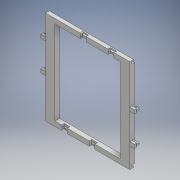
# Autodesk Inventor part: Male_Final
Saved by Autodesk Inventor 2017 (Build 210142000, 142)
## iProperties
Created: 2018-11-19
Part Number: Male_Final
Material: Generic
Document SubType Name: Modeling
Designer: Ralph
Density: 1 g/cm^3
Appearance: Default
Author: Ralph
Autodesk Inventor part; units mm, degrees
ref_plane "YZ Plane" through (0, 0, 0) normal (1, 0, 0) x (0, 1, 0)
ref_plane "XZ Plane" through (0, 0, 0) normal (0, 1, 0) x (-1, 0, 0)
ref_plane "XY Plane" through (0, 0, 0) normal (0, 0, 1) x (1, 0, 0)
sketch "Sketch1" plane through (0, 0, 0) normal (0, 1, 0) x (-1, 0, 0)
  line L0 (0, 0) -> (90, 0)
  line L1 (90, 0) -> (90, -100)
  line L2 (90, -100) -> (0, -100)
  line L3 (0, -100) -> (0, 0)
  line L4 (10, -5) -> (80, -5)
  line L5 (80, -5) -> (80, -95)
  line L6 (80, -95) -> (10, -95)
  line L7 (10, -95) -> (10, -5)
  line L8 (10, 0) -> (10, -5)
  line L9 (0, -5) -> (10, -5)
  dimension "d0" = 90
  dimension "d1" = 100
  dimension "d2" = 70
  dimension "d3" = 90
  dimension "d4" = 5
  dimension "d5" = 10
  constraints: 20 end point, 4 parallel, 3 perpendicular, 2 horizontal, 2 point on line, 1 vertical
  measures "d0" distance of L1.end L2.end
  measures "d1" distance of L0.end L1.end
  measures "d2" distance of L5.end L6.end
  measures "d3" distance of L4.end L5.end
  measures "d4" distance of L8.start L4.start
  measures "d5" distance of L9.start L4.start
extrude "Extrusion1" add sketch "Sketch1" along normal blind 5
sketch "Sketch2" plane through (0, 5, 0) normal (0, 1, 0) x (1, 0, 0)
  line L0 (0, 0) -> (0, 100) projected
  line L1 (0, 0) -> (0, 1.5)
  line L2 (0, 1.5) -> (0, 3)
  line L3 (0, 1.5) -> (-90, 1.5)
  line L4 (-90, 1.5) -> (-90, 3)
  line L5 (-90, 3) -> (0, 3)
  line L6 (0, 3) -> (0, 1.5)
  line L7 (0, 0) -> (0, 97)
  line L8 (0, 97) -> (0, 98.5)
  line L9 (0, 97) -> (-90, 97)
  line L10 (-90, 97) -> (-90, 98.5)
  line L11 (-90, 98.5) -> (0, 98.5)
  line L12 (0, 98.5) -> (0, 97)
  line L13 (0, 1.5) -> (0, 1.25)
  line L14 (0, 1.25) -> (0, 3.25)
  line L15 (0, 1.25) -> (-90, 1.25)
  line L16 (-90, 1.25) -> (-90, 3.25)
  line L17 (-90, 3.25) -> (0, 3.25)
  line L18 (0, 3.25) -> (0, 1.25)
  line L19 (0, 98.5) -> (0, 98.75)
  line L20 (0, 98.75) -> (0, 96.75)
  line L21 (0, 96.75) -> (-90, 96.75)
  line L22 (-90, 96.75) -> (-90, 98.75)
  line L23 (-90, 98.75) -> (0, 98.75)
  line L24 (0, 98.75) -> (0, 96.75)
  dimension "d8" = 1.5
  dimension "d9" = 1.5
  dimension "d10" = 90
  dimension "d11" = 1.5
  dimension "d12" = 97
  dimension "d13" = 1.5
  dimension "d14" = 90
  dimension "d15" = 1.5
  dimension "d16" = 0.25
  dimension "d17" = 2
  dimension "d18" = 90
  dimension "d19" = 2
  dimension "d20" = 0.25
  dimension "d21" = 2
  dimension "d22" = 90
  dimension "d23" = 2
  constraints: 48 end point, 8 parallel, 8 point on line, 4 horizontal, 4 perpendicular
  measures "d8" distance of L0.start L1.end
  measures "d9" distance of L1.end L2.end
  measures "d10" distance of L4.end L5.end
  measures "d11" distance of L3.end L4.end
  measures "d12" distance of L0.start L7.end
  measures "d13" distance of L7.end L8.end
  measures "d14" distance of L10.end L11.end
  measures "d15" distance of L9.end L10.end
  measures "d16" distance of L1.end L13.end
  measures "d17" distance of L13.end L14.end
  measures "d18" distance of L16.end L17.end
  measures "d19" distance of L15.end L16.end
  measures "d20" distance of L11.end L19.end
  measures "d21" distance of L19.end L20.end
  measures "d22" distance of L22.end L23.end
  measures "d23" distance of L21.end L22.end
extrude "Extrusion2" cut sketch "Sketch2" against normal blind 2.75
sketch "Sketch3" plane through (0, 0, -100) normal (0, 0, -1) x (-1, 0, 0)
  line L0 (90, 0) -> (0, 0) projected
  line L1 (0, 0) -> (35, 0)
  line L2 (35, 0) -> (45, 0)
  line L3 (80, 0) -> (10, 0) projected
  line L4 (45, 0) -> (65, 0)
  line L5 (65, 0) -> (75, 0)
  line L6 (35, 0) -> (38, 0)
  line L7 (38, 0) -> (37.75, 0)
  line L8 (37.75, 0) -> (43.25, 0)
  line L9 (43.25, 0) -> (43, 0)
  line L10 (37.75, 0) -> (37.75, 2.75)
  line L11 (37.75, 2.75) -> (43.25, 2.75)
  line L12 (43.25, 2.75) -> (43.25, 0)
  line L13 (75, 0) -> (72, 0)
  line L14 (72, 0) -> (72.25, 0)
  line L15 (72.25, 0) -> (66.75, 0)
  line L16 (66.75, 0) -> (66.75, 2.75)
  line L17 (66.75, 2.75) -> (72.25, 2.75)
  line L18 (72.25, 2.75) -> (72.25, 0)
  dimension "d26" = 35
  dimension "d27" = 10
  dimension "d28" = 20
  dimension "d29" = 10
  dimension "d30" = 3
  dimension "d31" = 0.25
  dimension "d32" = 5.5
  dimension "d33" = 0.25
  dimension "d34" = 2.75
  dimension "d35" = 3
  dimension "d36" = 0.25
  dimension "d37" = 5.5
  dimension "d38" = 2.75
  constraints: 34 end point, 12 point on line, 4 perpendicular, 1 midpoint
  measures "d26" distance of L0.end L1.end
  measures "d27" distance of L1.end L2.end
  measures "d28" distance of L2.end L4.end
  measures "d29" distance of L4.end L5.end
  measures "d30" distance of L1.end L6.end
  measures "d31" distance of L6.end L7.end
  measures "d32" distance of L7.end L8.end
  measures "d33" distance of L8.end L9.end
  measures "d34" distance of L7.end L10.end
  measures "d35" distance of L5.end L13.end
  measures "d36" distance of L13.end L14.end
  measures "d37" distance of L14.end L15.end
  measures "d38" distance of L15.end L16.end
extrude "Extrusion3" cut sketch "Sketch3" against normal blind 3
sketch "Sketch6" plane through (-90, 0, 0) normal (0, 0, 1) x (1, 0, 0)
  line L0 (0, 0) -> (0, 5) projected
  line L1 (0, 0) -> (35, 0)
  line L2 (17.75, 0) -> (0, 0) projected
  line L3 (35, 0) -> (45, 0)
  line L4 (45, 0) -> (65, 0)
  line L5 (80, 0) -> (10, 0) projected
  line L6 (65, 0) -> (75, 0)
  line L7 (75, 0) -> (72, 0)
  line L8 (72, 0) -> (72.25, 0)
  line L9 (72.25, 0) -> (66.75, 0)
  line L10 (66.75, 0) -> (66.75, 2.75)
  line L11 (66.75, 2.75) -> (72.25, 2.75)
  line L12 (72.25, 2.75) -> (72.25, 0)
  line L13 (35, 0) -> (38, 0)
  line L14 (38, 0) -> (37.75, 0)
  line L15 (37.75, 0) -> (43.25, 0)
  line L16 (43.25, 0) -> (43.25, 2.75)
  line L17 (43.25, 2.75) -> (37.75, 2.75)
  line L18 (37.75, 2.75) -> (37.75, 0)
  point P0 (90, 0)
  dimension "d45" = 35
  dimension "d46" = 10
  dimension "d47" = 20
  dimension "d48" = 10
  dimension "d49" = 3
  dimension "d50" = 0.25
  dimension "d51" = 5.5
  dimension "d52" = 2.75
  dimension "d53" = 3
  dimension "d54" = 0.25
  dimension "d55" = 5.5
  dimension "d56" = 2.75
  constraints: 32 end point, 12 point on line, 4 perpendicular
  measures "d45" distance of L0.start L1.end
  measures "d46" distance of L1.end L3.end
  measures "d47" distance of L3.end L4.end
  measures "d48" distance of L4.end L6.end
  measures "d49" distance of L6.end L7.end
  measures "d50" distance of L7.end L8.end
  measures "d51" distance of L8.end L9.end
  measures "d52" distance of L9.end L10.end
  measures "d53" distance of L1.end L13.end
  measures "d54" distance of L13.end L14.end
  measures "d55" distance of L14.end L15.end
  measures "d56" distance of L15.end L16.end
extrude "Extrusion4" cut sketch "Sketch6" against normal blind 3
sketch "Sketch7" plane through (0, 0, 0) normal (0, -1, 0) x (1, 0, 0)
  line L0 (-43.25, -100) -> (-43.25, -98.75) projected
  line L1 (-43.25, -97) -> (-37.25, -97)
  line L2 (-37.25, -97) -> (-37.25, -94.75)
  line L3 (-37.25, -94.75) -> (-43.25, -94.75)
  line L4 (-43.25, -94.75) -> (-43.25, -97)
  line L5 (-66.75, -100) -> (-66.75, -98.75) projected
  line L6 (-66.75, -97) -> (-72.75, -97)
  line L7 (-72.75, -97) -> (-72.75, -94.75)
  line L8 (-72.75, -94.75) -> (-66.75, -94.75)
  line L9 (-66.75, -94.75) -> (-66.75, -97)
  line L10 (-17.75, -3) -> (-23.25, -3) projected
  line L11 (-23.25, -3) -> (-17.25, -3)
  line L12 (-17.25, -3) -> (-17.25, -5.25)
  line L13 (-17.25, -5.25) -> (-23.25, -5.25)
  line L14 (-23.25, -5.25) -> (-23.25, -3)
  line L15 (-46.75, -3) -> (-52.25, -3) projected
  line L16 (-46.75, -3) -> (-52.75, -3)
  line L17 (-52.75, -3) -> (-52.75, -5.25)
  line L18 (-52.75, -5.25) -> (-46.75, -5.25)
  line L19 (-46.75, -5.25) -> (-46.75, -3)
  point P0 (0, 0)
  dimension "d71" = 6
  dimension "d72" = 2.25
  dimension "d73" = 6
  dimension "d74" = 2.25
  dimension "d75" = 6
  dimension "d76" = 2.25
  dimension "d77" = 6
  dimension "d78" = 2.25
  constraints: 32 end point, 8 parallel, 4 horizontal, 4 perpendicular
  measures "d71" distance of L3.end L2.end
  measures "d72" distance of L2.end L1.end
  measures "d73" distance of L7.end L8.end
  measures "d74" distance of L6.end L7.end
  measures "d75" distance of L12.end L13.end
  measures "d76" distance of L11.end L12.end
  measures "d77" distance of L18.end L17.end
  measures "d78" distance of L17.end L16.end
extrude "Extrusion5" cut sketch "Sketch7" against normal blind 2.75
fillet "Fillet1" radius 1 4 edges at (-52.25, 1.375, 0) (-17.75, 1.375, 0) (-37.75, 1.375, -100) (-72.25, 1.375, -100)
sketch "Sketch9" plane through (-90, 0, -100) normal (-1, 0, 0) x (0, 0, 1)
  line L0 (0, 0) -> (0, 5) projected
  line L1 (0, 5) -> (40, 5)
  line L2 (3.25, 5) -> (96.75, 5) projected
  line L3 (40, 5) -> (50, 5)
  line L4 (50, 5) -> (70, 5)
  line L5 (70, 5) -> (80, 5)
  line L6 (80, 5) -> (80, 2.5)
  line L7 (80, 2.5) -> (0, 2.5)
  line L8 (0, 2.5) -> (0, 5)
  line L9 (80, 5) -> (77, 5)
  line L10 (77, 5) -> (77, 2.5)
  line L11 (77, 5) -> (75, 5)
  line L12 (75, 5) -> (75, 2.5)
  line L13 (40, 5) -> (43, 5)
  line L14 (43, 5) -> (45, 5)
  line L15 (45, 5) -> (45, 2.5)
  line L16 (43, 5) -> (43, 2.5)
  line L17 (43, 5) -> (45, 5)
  line L18 (45, 5) -> (45, 2.5)
  line L19 (45, 2.5) -> (43, 2.5)
  line L20 (43, 2.5) -> (43, 5)
  point P0 (100, 0)
  dimension "d85" = 40
  dimension "d86" = 10
  dimension "d87" = 20
  dimension "d88" = 10
  dimension "d89" = 2.5
  dimension "d91" = 3
  dimension "d92" = 2
  dimension "d93" = 3
  dimension "d94" = 2
  constraints: 38 end point, 9 point on line, 8 perpendicular, 3 midpoint, 2 parallel, 1 horizontal
  measures "d85" distance of L0.end L1.end
  measures "d86" distance of L1.end L3.end
  measures "d87" distance of L3.end L4.end
  measures "d88" distance of L4.end L5.end
  measures "d89" distance of L5.end L6.end
  measures "d91" distance of L5.end L9.end
  measures "d92" distance of L9.end L11.end
  measures "d93" distance of L1.end L13.end
  measures "d94" distance of L13.end L14.end
extrude "Extrusion6" add sketch "Sketch9" along normal blind 3 contours L16 L2 L15 L7 | L12 L2 L10 L7
fillet "Fillet2" radius 1 4 edges at (-90, 3.75, -23) (-90, 3.75, -25) (-90, 3.75, -55) (-90, 3.75, -57)
sketch "Sketch10" plane through (-93, 0, -100) normal (-1, 0, 0) x (0, 0, 1)
  line L0 (75, 2.5) -> (77, 2.5) projected
  line L1 (75, 2.5) -> (77.75, 2.5)
  line L2 (77.75, 2.5) -> (77.75, 5)
  line L3 (77.75, 5) -> (75, 5)
  line L4 (75, 5) -> (75, 2.5)
  line L5 (45, 2.5) -> (45, 5) projected
  line L6 (45, 2.5) -> (42.25, 2.5)
  line L7 (42.25, 2.5) -> (42.25, 5)
  line L8 (42.25, 5) -> (45, 5)
  line L9 (45, 5) -> (45, 2.5)
  point P0 (100, 0)
  dimension "d98" = 2.75
  dimension "d99" = 2.5
  dimension "d100" = 2.75
  dimension "d101" = 2.5
  constraints: 16 end point, 4 parallel, 2 horizontal, 2 perpendicular
  measures "d98" distance of L3.end L2.end
  measures "d99" distance of L2.end L1.end
  measures "d100" distance of L7.end L8.end
  measures "d101" distance of L6.end L7.end
extrude "Extrusion7" add sketch "Sketch10" along normal blind 2
sketch "Sketch12" plane through (0, 0, 0) normal (1, 0, 0) x (0, 0, -1)
  line L0 (0, 0) -> (0, 5) projected
  line L1 (0, 5) -> (40, 5)
  line L2 (5, 5) -> (95, 5) projected
  line L3 (40, 5) -> (50, 5)
  line L4 (50, 5) -> (70, 5)
  line L5 (70, 5) -> (80, 5)
  line L6 (80, 5) -> (80, 2.5)
  line L7 (95, 0) -> (5, 0) projected
  line L8 (80, 2.5) -> (0, 2.5)
  line L9 (0, 2.5) -> (0, 5)
  line L10 (80, 5) -> (77, 5)
  line L11 (77, 5) -> (75, 5)
  line L12 (75, 5) -> (75, 2.5)
  line L13 (77, 5) -> (77, 2.5)
  line L14 (77, 2.5) -> (75, 2.5)
  line L15 (40, 5) -> (43, 5)
  line L16 (54, 5) -> (26, 5) projected
  line L17 (43, 5) -> (45, 5)
  line L18 (45, 5) -> (45, 2.5)
  line L19 (43, 5) -> (43, 2.5)
  line L20 (43, 2.5) -> (45, 2.5)
  dimension "d105" = 40
  dimension "d106" = 10
  dimension "d107" = 20
  dimension "d108" = 10
  dimension "d109" = 2.5
  dimension "d110" = 3
  dimension "d111" = 2
  dimension "d112" = 3
  dimension "d113" = 2
  constraints: 34 end point, 10 point on line, 7 perpendicular, 2 collinear, 2 midpoint
  measures "d105" distance of L0.end L1.end
  measures "d106" distance of L1.end L3.end
  measures "d107" distance of L3.end L4.end
  measures "d108" distance of L4.end L5.end
  measures "d109" distance of L5.end L6.end
  measures "d110" distance of L5.end L10.end
  measures "d111" distance of L10.end L11.end
  measures "d112" distance of L1.end L15.end
  measures "d113" distance of L15.end L17.end
extrude "Extrusion8" add sketch "Sketch12" along normal blind 3 contours L19 L2 L18 L8 | L12 L2 L13 L8
fillet "Fillet3" radius 1 4 edges at (0, 3.75, -43) (0, 3.75, -45) (0, 3.75, -75) (0, 3.75, -77)
sketch "Sketch13" plane through (3, 0, 0) normal (1, 0, 0) x (0, 0, -1)
  line L0 (45, 5) -> (45, 2.5) projected
  line L1 (45, 2.5) -> (42.25, 2.5)
  line L2 (42.25, 2.5) -> (42.25, 5)
  line L3 (42.25, 5) -> (45, 5)
  line L4 (45, 5) -> (45, 2.5)
  line L5 (74, 2.5) -> (75, 2.5) projected
  line L6 (75, 2.5) -> (77.75, 2.5)
  line L7 (77.75, 2.5) -> (77.75, 5)
  line L8 (77.75, 5) -> (75, 5)
  line L9 (75, 5) -> (75, 2.5)
  point P0 (0, 0)
  dimension "d117" = 2.75
  dimension "d118" = 2.5
  dimension "d119" = 2.75
  dimension "d120" = 2.5
  constraints: 16 end point, 4 parallel, 2 horizontal, 2 perpendicular
  measures "d117" distance of L2.end L3.end
  measures "d118" distance of L1.end L2.end
  measures "d119" distance of L8.end L7.end
  measures "d120" distance of L7.end L6.end
extrude "Extrusion9" add sketch "Sketch13" along normal blind 2
sketch "Sketch11" plane through (0, 5, 0) normal (0, 1, 0) x (1, 0, 0)
  line L0 (-93, 22.25) -> (-95, 22.25) projected
  line L1 (-93, 22.25) -> (-92.25, 22.25)
  line L2 (-93, 57.75) -> (-93, 57) projected
  line L3 (-93, 57.75) -> (-92.25, 57.75)
  line L4 (3, 43) -> (3, 42.25) projected
  line L5 (3, 42.25) -> (2.25, 42.25)
  line L6 (3, 77.75) -> (3, 77) projected
  line L7 (3, 77.75) -> (2.25, 77.75)
  point P0 (0, 0)
  dimension "d104" = 0.75
  dimension "d123" = 0.75
  dimension "d124" = 0.75
  constraints: 8 end point, 4 horizontal
  measures "d104" distance of L0.start L1.end
  measures "d123" distance of L4.end L5.end
  measures "d124" distance of L6.start L7.end
hole "Hole1" at (2.25, 5, -42.25) at (2.25, 5, -77.75) at (-92.25, 5, -22.25) at (-92.25, 5, -57.75) direction (0, -1, 0) diameter 2.125 end through all
chamfer "Chamfer1" distance 1 distance2 1.25 1 edges at (5, 3.75, -42.25) measured on face at (5, 3.3333, -44.0833)
chamfer "Chamfer2" distance 1 distance2 1.25 1 edges at (5, 3.75, -77.75) measured on face at (5, 4.1667, -75.9167)
chamfer "Chamfer3" distance 1 distance2 1.25 1 edges at (-95, 3.75, -57.75) measured on face at (-95, 3.3333, -55.9167)
chamfer "Chamfer4" distance 1 distance2 1.25 1 edges at (-95, 3.75, -22.25) measured on face at (-95, 4.1667, -24.0833)
sketch "Sketch14" plane through (0, 5, 0) normal (0, 1, 0) x (1, 0, 0)
  line L0 (-52.25, 1.25) -> (-90, 1.25) projected
  line L1 (0, 0) -> (-90, 0)
  line L2 (-90, 0) -> (-90, 1.25)
  line L3 (-90, 1.25) -> (0, 1.25)
  line L4 (0, 1.25) -> (0, 0)
  line L5 (-37.75, 98.75) -> (0, 98.75) projected
  line L6 (-90, 100) -> (-90, 0) projected
  line L7 (0, 98.75) -> (-90, 98.75)
  line L8 (-90, 98.75) -> (-90, 100)
  line L9 (-90, 100) -> (0, 100)
  line L10 (0, 100) -> (0, 98.75)
  constraints: 16 end point, 4 parallel, 2 horizontal, 2 perpendicular
extrude "Extrusion10" cut sketch "Sketch14" against normal blind 1
sketch "Sketch15" plane through (0, 0, 0) normal (0, -1, 0) x (1, 0, 0)
  point P0 (0, 0)
sketch "Sketch16" plane through (0, 0, 0) normal (0, -1, 0) x (1, 0, 0)
  line L0 (-90, -100) -> (0, -100) projected
  line L1 (0, -100) -> (0, -80)
  line L2 (0, 0) -> (0, -100) projected
  line L3 (0, -80) -> (0, -70)
  line L4 (0, -70) -> (0, -50)
  line L5 (0, -50) -> (0, -40)
  line L6 (0, -3.25) -> (0, -42) projected
  line L7 (0, -40) -> (0, -42)
  line L8 (0, -42) -> (5, -42)
  line L9 (5, -42) -> (5, -46)
  arc A0 (1, -45) -> (0, -46) centre (1, -46) ccw projected
  line L10 (5, -46) -> (0, -46)
  line L11 (0, -46) -> (0, -42)
  line L12 (0, -42) -> (0.25, -42)
  line L13 (0.25, -42) -> (0.25, -46)
  line L14 (0, -80) -> (0, -78)
  line L15 (0, -78) -> (0, -74)
  line L16 (0, -74) -> (5, -74)
  line L17 (5, -74) -> (5, -78)
  line L18 (5, -78) -> (0, -78)
  line L19 (0, -78) -> (0.25, -78)
  line L20 (0.25, -78) -> (0.25, -74)
  line L21 (0, 0) -> (-90, 0) projected
  line L22 (-90, 0) -> (-90, -20)
  line L23 (-72.75, -96.75) -> (-90, -96.75) projected
  line L24 (-90, -20) -> (-90, -30)
  line L25 (-90, -30) -> (-90, -50)
  line L26 (-90, -50) -> (-90, -60)
  line L27 (-90, -20) -> (-90, -22)
  line L28 (-90, -100) -> (-90, 0) projected
  line L29 (-90, -22) -> (-95, -22)
  line L30 (-95, -22) -> (-95, -26)
  line L31 (-95, -26) -> (-90, -26)
  line L32 (-90, -26) -> (-90, -22)
  line L33 (-90, -22) -> (-90.25, -22)
  line L34 (-90.25, -22) -> (-90.25, -26)
  line L35 (-90, -96.75) -> (-90, -58) projected
  line L36 (-90, -60) -> (-90, -58)
  line L37 (-90, -58) -> (-95, -58)
  line L38 (-95, -58) -> (-95, -54)
  line L39 (-95, -54) -> (-90, -54)
  line L40 (-90, -54) -> (-90, -58)
  line L41 (-90, -54) -> (-90.25, -54)
  line L42 (-90.25, -54) -> (-90.25, -58)
  dimension "d146" = 20
  dimension "d147" = 10
  dimension "d148" = 20
  dimension "d149" = 10
  dimension "d150" = 5
  dimension "d151" = 4
  dimension "d152" = 0.25
  dimension "d153" = 2
  dimension "d154" = 4
  dimension "d155" = 5
  dimension "d156" = 4
  dimension "d157" = 0.25
  dimension "d158" = 20
  dimension "d159" = 10
  dimension "d160" = 20
  dimension "d161" = 10
  dimension "d162" = 2
  dimension "d163" = 5
  dimension "d164" = 4
  dimension "d165" = 0.25
  dimension "d166" = 2
  dimension "d167" = 5
  dimension "d168" = 4
  dimension "d169" = 0.25
  constraints: 72 end point, 15 point on line, 9 perpendicular, 4 parallel, 3 horizontal, 2 vertical, 1 collinear, 1 tangent, 5 other
  measures "d146" distance of L0.end L1.end
  measures "d147" distance of L1.end L3.end
  measures "d148" distance of L3.end L4.end
  measures "d149" distance of L4.end L5.end
  measures "d150" distance of L6.end L8.end
  measures "d151" distance of L8.end L9.end
  measures "d152" distance of L6.end L12.end
  measures "d153" distance of L1.end L14.end
  measures "d154" distance of L14.end L15.end
  measures "d155" distance of L15.end L16.end
  measures "d156" distance of L16.end L17.end
  measures "d157" distance of L14.end L19.end
  measures "d158" distance of L21.end L22.end
  measures "d159" distance of L22.end L24.end
  measures "d160" distance of L24.end L25.end
  measures "d161" distance of L25.end L26.end
  measures "d162" distance of L22.end L27.end
  measures "d163" distance of L31.end L30.end
  measures "d164" distance of L30.end L29.end
  measures "d165" distance of L27.end L33.end
  measures "d166" distance of L26.end L35.end
  measures "d167" distance of L38.end L39.end
  measures "d168" distance of L37.end L38.end
  measures "d169" distance of L39.end L41.end
extrude "Extrusion11" add sketch "Sketch16" against normal blind 2.3 contours L20 L16 L17 L18 | L37 L38 L39 L42 | L13 L8 L9 L10 | L31 L30 L29 L34
body "Solid1"
